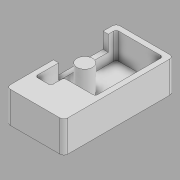
# Autodesk Inventor part: Lab8A01209499P1
Saved by Autodesk Inventor 2020 (Build 240168000, 168)
## iProperties
Created: 2019-10-04
Part Number: Lab8A01209499P1
Material: Genérico
Document SubType Name: Modeling
Designer: gerar
Density: 1 g/cm^3
Appearance: Valor por defecto
Author: gerar
Autodesk Inventor part; units mm, degrees
ref_plane "YZ Plane" through (0, 0, 0) normal (1, 0, 0) x (0, 1, 0)
ref_plane "XZ Plane" through (0, 0, 0) normal (0, 1, 0) x (-1, 0, 0)
ref_plane "XY Plane" through (0, 0, 0) normal (0, 0, 1) x (1, 0, 0)
sketch "Boceto1" plane through (0, 0, 0) normal (0, 1, 0) x (-1, 0, 0)
  line L0 (30.1625, 61.9125) -> (-30.1625, 61.9125) construction
  line L1 (-30.1625, 61.9125) -> (-30.1625, -61.9125) construction
  line L2 (-30.1625, -61.9125) -> (30.1625, -61.9125) construction
  line L3 (30.1625, -61.9125) -> (30.1625, 61.9125) construction
  line L4 (30.1625, 61.9125) -> (-30.1625, -61.9125) construction
  line L5 (-30.1625, 61.9125) -> (30.1625, -61.9125) construction
  arc A0 (-34.925, -61.9125) -> (-30.1625, -66.675) centre (-30.1625, -61.9125) ccw
  arc A1 (-30.1625, 66.675) -> (-34.925, 61.9125) centre (-30.1625, 61.9125) ccw
  arc A2 (34.925, 61.9125) -> (30.1625, 66.675) centre (30.1625, 61.9125) ccw
  line L6 (34.925, -61.9125) -> (34.925, 61.9125)
  line L7 (30.1625, 66.675) -> (-30.1625, 66.675)
  line L8 (-34.925, 61.9125) -> (-34.925, -61.9125)
  line L9 (30.1625, -66.675) -> (-30.1625, -66.675)
  arc A3 (30.1625, -66.675) -> (34.925, -61.9125) centre (30.1625, -61.9125) ccw
  arc A4 (30.1625, -57.15) -> (28.0767, -57.6311) centre (30.1625, -61.9125) ccw
  point P0 (0, 0)
  dimension "d0" = 60.325
  dimension "d1" = 123.825
  dimension "d3" = 9.525
  dimension "d4" = 9.525
  dimension "d5" = 9.525
  dimension "d6" = 69.85
  dimension "d7" = 133.35
  constraints: 20 end point, 10 point on circle, 5 centre point, 4 coincident, 4 tangent, 3 horizontal, 2 midpoint, 2 parallel, 2 point on line, 2 vertical, 1 perpendicular
  measures "d0" distance of L2.end L1.end
  measures "d1" distance between parallel lines of L0 L2
  measures "d3" diameter of A0
  measures "d4" diameter of A1
  measures "d5" diameter of A2
  measures "d6" distance between parallel lines of L8 L6
  measures "d7" distance between parallel lines of L7 L9
extrude "Extrusión1" add sketch "Boceto1" along normal blind 38.1
sketch "Boceto3" plane through (0, 38.1, 0) normal (0, 1, 0) x (1, 0, 0)
  line L0 (-25.4, 60.325) -> (25.4, 60.325)
  line L1 (28.575, 57.15) -> (28.575, -19.05)
  line L2 (25.4, -22.225) -> (-6.35, -22.225)
  line L3 (-9.525, -25.4) -> (-9.525, -34.925)
  line L4 (-28.575, 57.15) -> (-28.575, -34.925)
  line L5 (-25.4, -38.1) -> (-12.7, -38.1)
  line L6 (30.1625, 66.675) -> (-30.1625, 66.675) projected
  line L7 (-34.925, 61.9125) -> (-34.925, -61.9125) projected
  line L8 (34.925, -61.9125) -> (34.925, 61.9125) projected
  line L9 (-30.1625, -66.675) -> (30.1625, -66.675) projected
  arc A0 (-25.4, 60.325) -> (-28.575, 57.15) centre (-25.4, 57.15) ccw
  arc A1 (28.575, 57.15) -> (25.4, 60.325) centre (25.4, 57.15) ccw
  arc A2 (25.4, -22.225) -> (28.575, -19.05) centre (25.4, -19.05) ccw
  arc A3 (-6.35, -22.225) -> (-9.525, -25.4) centre (-6.35, -25.4) ccw
  arc A4 (-12.7, -38.1) -> (-9.525, -34.925) centre (-12.7, -34.925) ccw
  arc A5 (-28.575, -34.925) -> (-25.4, -38.1) centre (-25.4, -34.925) ccw
  point P0 (0, 0)
  dimension "d20" = 6.35
  dimension "d21" = 6.35
  dimension "d22" = 6.35
  dimension "d23" = 44.45
  dimension "d24" = 15.875
  dimension "d25" = 38.1
  dimension "d26" = 3.175
  constraints: 12 end point, 12 point on circle, 12 tangent, 6 centre point, 5 equal radius, 4 perpendicular, 1 horizontal, 1 vertical
  measures "d20" distance between parallel lines of L0 L6
  measures "d21" distance between parallel lines of L7 L4
  measures "d22" distance between parallel lines of L8 L1
  measures "d23" distance between parallel lines of L9 L2
  measures "d24" distance between parallel lines of L2 L5
  measures "d25" distance between parallel lines of L1 L3
  measures "d26" radius of A0
extrude "Extrusión2" cut sketch "Boceto3" against normal blind 31.75
sketch "Boceto4" plane through (-34.925, 0, -61.9125) normal (-1, 0, 0) x (0, 0, 1)
  line L0 (11.1125, 38.1) -> (71.4166, 38.1)
  line L1 (71.4166, 38.1) -> (71.4166, 20.6375)
  line L2 (69.8291, 19.05) -> (11.1125, 19.05)
  line L3 (11.1125, 19.05) -> (11.1125, 38.1)
  line L4 (-4.7625, 0) -> (-4.7625, 38.1) projected
  line L5 (0, 38.1) -> (123.825, 38.1) projected
  arc A0 (69.8291, 19.05) -> (71.4166, 20.6375) centre (69.8291, 20.6375) ccw
  point P0 (61.9125, 0)
  dimension "d29" = 15.875
  dimension "d30" = 19.05
  dimension "d31" = 60.325
  dimension "d32" = 3.175
  constraints: 8 end point, 2 parallel, 2 point on circle, 2 tangent, 1 centre point, 1 collinear, 1 horizontal, 1 perpendicular
  measures "d29" distance between parallel lines of L4 L3
  measures "d30" distance between parallel lines of L0 L2
  measures "d31" distance of L1.end L2.end
  measures "d32" diameter of A0
extrude "Extrusión3" cut sketch "Boceto4" against normal blind 6.35
sketch "Boceto6" plane through (0, 0, 0) normal (0, -1, 0) x (1, 0, 0)
  circle A0 centre (-12.7, -6.35) radius 9.525
  line L0 (30.1625, -66.675) -> (-30.1625, -66.675) projected
  line L1 (-34.925, -61.9125) -> (-34.925, 61.9125) projected
  point P0 (0, 0)
  dimension "d44" = 19.05
  dimension "d45" = 60.325
  dimension "d46" = 22.225
  constraints: 1 centre point
  measures "d44" diameter of A0
  measures "d45" distance from line of L0 A0.centre
  measures "d46" distance from line of L1 A0.centre
extrude "Extrusión5" add sketch "Boceto6" against normal blind 38.1
sketch "Boceto7" plane through (0, 0, 0) normal (0, -1, 0) x (1, 0, 0)
  circle A0 centre (-12.7, -6.35) radius 9.525 construction
  line L0 (28.575, -57.15) -> (28.575, 19.05) construction
  arc A1 (28.575, 19.05) -> (25.4, 22.225) centre (25.4, 19.05) ccw construction
  line L1 (25.4, 22.225) -> (-6.35, 22.225) construction
  line L2 (-9.525, 25.4) -> (-9.525, 34.925) construction
  arc A2 (-9.525, 25.4) -> (-6.35, 22.225) centre (-6.35, 25.4) ccw construction
  arc A3 (-9.525, 34.925) -> (-12.7, 38.1) centre (-12.7, 34.925) ccw construction
  line L3 (-12.7, 38.1) -> (-25.4, 38.1) construction
  arc A4 (-25.4, 38.1) -> (-28.575, 34.925) centre (-25.4, 34.925) ccw construction
  line L4 (-28.575, 34.925) -> (-28.575, -57.15) construction
  line L5 (-25.4, -60.325) -> (25.4, -60.325) construction
  arc A5 (25.4, -60.325) -> (28.575, -57.15) centre (25.4, -57.15) ccw construction
  arc A6 (-28.575, -57.15) -> (-25.4, -60.325) centre (-25.4, -57.15) ccw construction
  point P0 (0, 0)
